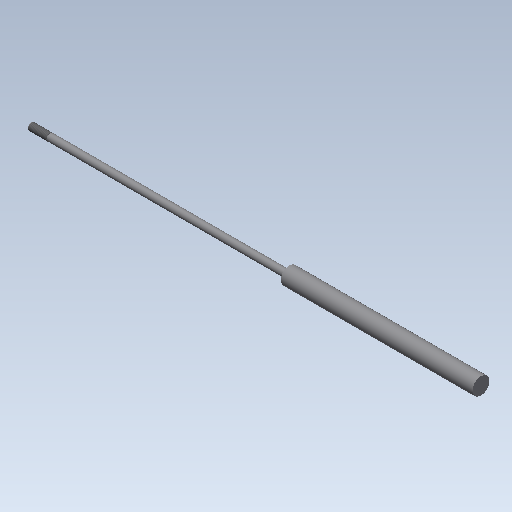
# Autodesk Inventor part: 015.5-P0000_rod
Saved by Autodesk Inventor 2020 (Build 240168000, 168)
## iProperties
Created: 2020-01-07
Part Number: 015.5-P0000_rod
Material: Generic
Catalog Web Link: www.cadenas.de
Description: Standard Air Cylinder_rod-Original Line - Standard Air Cylinders
Vendor: BIMBA
Document SubType Name: Modeling
Designer: psadmin
Manufacturer: BIMBA
Mass: 15.5246 g
Surface Area: 71.9082 cm^2
Volume: 15.5246 cm^3
Density: 1 g/cm^3
Appearance: PSOLRGB-181-181-181
Category: PARTsolutions
Company: BIMBA
PSOL_IDENT_0: {$CADENAS_DATA\23d-libs\bimba\bimba_brand\bimba_imperial\bimba_full_line\original_line_cylinders\sta
PSOL_IDENT_1: ndard_air_cylinders\rod.prj},331 {VTYP=3D},{NB=015.5-P0000_rod},{LINA=015.5-P0000_rod},{NN=Standard
PSOL_IDENT_2: Air Cylinder_rod},{DATE=23.12.2019 10:36:48},{GEOMDATE=27.08.2019 11:00:52},{VERSION=},{LINEID=30},{
PSOL_IDENT_3: WBVAR=STROKE,ACTING,MNT,DER,NR,BM,CO,M,EE,EEL,K,Q,Y,F,G,T,B,H,SER,SR,NT,W,E,HL,ST,STP,PRC,PB,COLOR1,
PSOL_IDENT_4: FCD,RCD,BCD,ZHJ},{WBNUMERIC=STROKE,EEL,COLOR1,FCD,RCD,BCD,ZHJ}  {NB=015.5-P0000_rod},{LINA=015.5-P00
PSOL_IDENT_5: 00_rod},{KT=DUMMY},{PN=015.5-P000},{DASH=-},{BORE=0.43750000},{BOREPN=01},{STROKE=5.500},{STROKEALG=
PSOL_IDENT_6: [0.001:50/0.001]},{STROKE1=5.500},{ACTING=},{ACTINGALG= '' , 'Single Acting' , 'R' , 'Reverse Single
PSOL_IDENT_7: Acting' , 'D' , 'Double Acting' },{ACTINGPN=},{MNT=P},{MNTALG= '' , 'Front Nose Mounting' , 'P' , '
PSOL_IDENT_8: Rear Pivot Mounting' , 'BF' , 'Front Block Mounting' , 'BR' , 'Rear Block Mounting for Vertical Posi
PSOL_IDENT_9: tioning' , 'BFT' , 'Front Block Trunnion Mounting' , 'BRT' , 'Rear Block Trunnion Mounting' },{TYPE=
PSOL_IDENT_10: },{MNTPN=P},{DER=},{DERALG= '' , 'N/A' },{NR=},{NRALG= '' , 'Standard' , 'NR' , 'Non-rotating - Hexa
PSOL_IDENT_11: gon Rod' },{NRPN=},{BM=},{BMALG= '' , 'N/A' },{BMPN=},{CO=},{COALG= '' , 'N/A' },{M=},{MALG= '', 'Wi
PSOL_IDENT_12: thout Magnet', 'M', 'With Magnet' },{EE=},{EEL=0},{EEMAX=44},{EEALG= '', 'Without Extra Extension', '
PSOL_IDENT_13: EE', 'With Extra Extension' },{EELALG=0},{EEPN=},{EEPN1=0.000},{K=},{KALG= '', 'Standard' , 'K' , 'P
PSOL_IDENT_14: orts Rotated 90deg' },{KPN=},{Q=},{QALG= '' , 'Without Side Ported Rear Head' , 'Q' , 'With Side Por
PSOL_IDENT_15: ted Rear Head' },{QPN=},{Y=},{YALG= '' , 'Without Pivot Bushing' , 'Y' , 'With Pivot Bushing' },{YPN=
PSOL_IDENT_16: },{F=},{FALG= '', 'Standard', 'F', 'Molycoated Body' },{FPN=},{G=},{GPN=},{T=},{TALG= '' , 'Standard'
PSOL_IDENT_17: , 'N' , 'Low Temperature' , 'V' , 'High Temperature' },{NPN=},{VPN=},{B=},{BALG= '', 'Without Bumpe
PSOL_IDENT_18: r' , 'B' , 'With Bumper' },{BPN=},{H=},{HALG= '', 'N/A' },{HPN=},{SER=},{SERALG= '' , 'N/A' },{SR=},
PSOL_IDENT_19: {SRALG= 'C' , 'Carbon Steel Rod' , 'SR' , '303 Stainless Steel Rod' , '' , '303 Stainless Steel Rod1'
PSOL_IDENT_20: },{SRPN=},{SRCON=0},{NT=},{NTPN=},{W=},{WALG= '' , 'N/A' },{WPN=},{E=},{EALG= '' , 'Without Special
PSOL_IDENT_21: Lube and Seals' , 'E' , 'With Special Lube and Seals' },{EPN=},{HL=},{HLALG= '' , 'N/A' },{ST=},{ST
PSOL_IDENT_22: ALG= '' , 'Without Switch Track' , 'T' , 'With Switch Track' },{STP=},{STPALG= '' , 'N/A' },{STPN=},
PSOL_IDENT_23: {PRC=},{PRCALG= '' , 'Without Piston Rod Clevis' , 'D-166-1' , 'With Piston Rod Clevis' },{PRCPN=},{
PSOL_IDENT_24: PB=},{PBALG= '' , 'Without Pivot Bracket' , 'D-167' , 'With Pivot Bracket' },{PBPN=},{TLEN=10.8620},
PSOL_IDENT_25: {TEXT=0.466667},{SPACE=0.266667},{FRAC=12.0900},{RGCON=},{RGDACCON=},{RHCON=P},{RHCONON=1},{RHACCON=
PSOL_IDENT_26: },{FNUTCON=0},{RNUTCON=0},{FNUTPN=},{RNUTPN=},{FNUTTRANS=0.0000},{RNUTTRANS=0.0000},{VHOLECON=2},{A1=
PSOL_IDENT_27: 0.6880},{A1N=0.6880},{A1P=1.1880},{A1B=1.1880},{A4=0.2500},{A4N=0.2500},{A4P=0.1880},{A5=0.0200},{A1
PSOL_IDENT_28: H=1.188},{A1NH=0.5000},{A1PH=1.1880},{A1BH=0.8120},{A1SH=0.0000},{A2H=0.1880},{A2NH=0.1880},{LENGTH=
PSOL_IDENT_29: 1.7500},{LENGTH1=1.7500},{LENGTH2=2.6100},{MUL=10.3400},{MUL11=10.3400},{MUL22=15.8400},{MUL33=10.34
PSOL_IDENT_30: 00},{MUL2=0.9400},{MUL211=0.9400},{MUL222=1.4400},{MUL233=0.9400},{SSS=11.0000},{RGLEN=0.4580},{RHLE
PSOL_IDENT_31: N=0.7700},{SSS1=11.0000},{A13=0.9380},{THDLEN1=0.5000},{THD1=0.1900},{TAB=UNF},{THDLEN=0.5000},{THD=
PSOL_IDENT_32: 0.1900},{OD=0.4465},{RODL=11.6520},{PL=4.9640},{RODDIA=0.1870},{HEX=0.1870},{RODTRANS=0.0000},{G1=0.
PSOL_IDENT_33: 0000},{ON=0},{G5=0.0000},{DERLEN=6.6880},{THOLE=0.0000},{WF=0.0000},{BADD=0.0000},{MADD=0.0000},{NVA
PSOL_IDENT_34: DD=0.000},{JRADD=0.00000},{COLOR=0.71,0.71,0.71,0.00},{GROOVE=1},{HOL=0},{D7=0.1590},{H1=0.0000},{D1=
PSOL_IDENT_35: 0.4840},{D1RH=0.7380},{D1P=0.0000},{D1B=0.7380},{D1N=0.4840},{D1NRH=0.4855},{D1BRH=0.4855},{D1PRH=0.
PSOL_IDENT_36: 7380},{BOZO=1},{HADD=0.000},{COLOR1=0},{DEFL=0.0000},{HEXL=0.0000},{SSADD=0.0000},{WFL=0.0000},{MOVE=
PSOL_IDENT_37: 0.0000},{PRCL2=0.37500},{PRCB=0.12000},{PRCTRANS=0.00000},{FCD=0},{RCD=0},{BCD=0},{ZHJ=0.000}
NN: Standard Air Cylinder_rod
NT: Standard
NB: 015.5-P0000_rod
NBSYN: $PN.$COLOR1._rod
LINA: 015.5-P0000_rod
PN: 015.5-P000
BORE: 0.4375
BOREPN: 01
STROKE: 5.5
ACTING: Single Acting
MNT: Rear Pivot Mounting
DER: N/A
NR: Standard
BM: N/A
CO: N/A
M: Without Magnet
EE: Without Extra Extension
EEL: 0
K: Standard
Q: Without Side Ported Rear Head
Y: Without Pivot Bushing
F: Standard
G: Without Magnalube Lubrication
T: Standard
B: Without Bumper
H: N/A
SER: N/A
SR: 303 Stainless Steel Rod1
W: N/A
E: Without Special Lube and Seals
HL: N/A
ST: Without Switch Track
STP: N/A
PRC: Without Piston Rod Clevis
PB: Without Pivot Bracket
A1N: 0.688
A1P: 1.188
A1B: 1.188
A4N: 0.25
A4P: 0.188
A5: 0.02
A1NH: 0.5
A1PH: 1.188
A1BH: 0.812
A1SH: 0
A2NH: 0.188
A13: 0.938
THDLEN1: 0.5
THD1: 0.19
TAB: UNF
OD: 0.4465
RODDIA: 0.187
HEX: 0.187
G1: 0
G5: 0
THOLE: 0
WF: 0
GROOVE: 1
D7: 0
D1P: 0
D1B: 0.738
D1N: 0.484
D1NRH: 0.4855
D1BRH: 0.4855
D1PRH: 0.738
COLOR1: 0
FCD: 0
RCD: 0
BCD: 0
ZHJ: 0
SUPPLIER: BIMBA
ARTICLENO: 015.5-P0000_rod
BOMINFO: 015.5-P0000_rod
CREATOR: CADENAS GmbH
d5: 0.000 in
d6: 0.000 in
d8: 0.000 in
d9: 0.000 in
d10: 0.000 in
Title: 015.5-P0000_rod
Author: Cadenas PARTsolutions
Comments: Original Line - Standard Air Cylinders
Autodesk Inventor part; units mm, degrees
sketch "Sketch_1" plane through (0, 0, 0) normal (0, 0, 1) x (1, 0, 0)
  line L0 (283.2608, 0) -> (0, 0)
  line L1 (0, 0) -> (0, 2.3749)
  line L2 (0, 2.3749) -> (157.1752, 2.3749)
  line L3 (157.1752, 2.3749) -> (157.1752, 5.6197)
  line L4 (157.1752, 5.6197) -> (283.2608, 5.6197)
  line L5 (283.2608, 5.6197) -> (283.2608, 0)
  line L6 (283.2608, 0) -> (0, 0)
  constraints: 14 end point
revolve "Revolution1" add sketch "Sketch_1" angle 360 about axis through (283.2608, 0, 0) along (1, 0, 0)
sketch "Sketch_3" plane through (0, 0, 0) normal (0, 0, 1) x (1, 0, 0)
  line L0 (0, 0) -> (-12.7, 0)
  line L1 (-12.7, 0) -> (-12.7, 1.9406)
  line L2 (-12.7, 1.9406) -> (-12.2276, 2.413)
  line L3 (-12.2276, 2.413) -> (0, 2.413)
  line L4 (0, 2.413) -> (0, 0)
  line L5 (0, 0) -> (-12.7, 0)
  constraints: 12 end point
revolve "Revolution2" add sketch "Sketch_3" angle 360 about axis through (0, 0, 0) along (1, 0, 0)
thread "Thread1" size "10-32 UNF" class "2A" standard "ANSI Unified Screw Threads" full length
sketch "Sketch_30" plane through (0, 0, 0) normal (0, 0, 1) x (1, 0, 0)
  line L0 (0, 0) -> (-0.254, 0)
  line L1 (-0.254, 2.159) -> (0, 2.159)
  line L2 (0, 2.159) -> (0, 2.667)
  line L3 (0, 2.667) -> (-0.254, 2.667)
  line L4 (-0.254, 2.667) -> (-0.254, 2.159)
  constraints: 10 end point
revolve "Revolution3" cut sketch "Sketch_30" angle 360 about axis through (0, 0, 0) along (1, 0, 0)
ref_plane "dia1_XY" through (0, 2.3749, 0) normal (1, 0, 0) x (0, 0, -1)
ref_plane "dia1_YZ" through (0, 2.3749, 0) normal (0, 0, -1) x (0, 1, 0)
ref_plane "dia1_ZX" through (0, 2.3749, 0) normal (0, 1, 0) x (1, 0, 0)
ref_plane "dia12_XY" through (0, 0, 6.1468) normal (1, 0, 0) x (0, 0, -1)
ref_plane "dia12_YZ" through (0, 0, 6.1468) normal (0, 0, -1) x (0, 1, 0)
ref_plane "dia12_ZX" through (0, 0, 6.1468) normal (0, 1, 0) x (1, 0, 0)
ref_plane "dia1r_XY" through (0, 0, 9.3726) normal (1, 0, 0) x (0, 0, -1)
ref_plane "dia1r_YZ" through (0, 0, 9.3726) normal (0, 0, -1) x (0, 1, 0)
ref_plane "dia1r_ZX" through (0, 0, 9.3726) normal (0, 1, 0) x (1, 0, 0)
ref_plane "dia2_XY" through (0, -2.3749, 0) normal (1, 0, 0) x (0, 0, -1)
ref_plane "dia2_YZ" through (0, -2.3749, 0) normal (0, 0, -1) x (0, 1, 0)
ref_plane "dia2_ZX" through (0, -2.3749, 0) normal (0, 1, 0) x (1, 0, 0)
ref_plane "dia22_XY" through (0, 0, -6.1468) normal (1, 0, 0) x (0, 0, -1)
ref_plane "dia22_YZ" through (0, 0, -6.1468) normal (0, 0, -1) x (0, 1, 0)
ref_plane "dia22_ZX" through (0, 0, -6.1468) normal (0, 1, 0) x (1, 0, 0)
ref_plane "dia2r_XY" through (0, 0, -9.3726) normal (1, 0, 0) x (0, 0, -1)
ref_plane "dia2r_YZ" through (0, 0, -9.3726) normal (0, 0, -1) x (0, 1, 0)
ref_plane "dia2r_ZX" through (0, 0, -9.3726) normal (0, 1, 0) x (1, 0, 0)
ref_plane "rl1_XY" through (-12.7, 0, 0) normal (1, 0, 0) x (0, 0, -1)
ref_plane "rl1_YZ" through (-12.7, 0, 0) normal (0, 0, -1) x (0, 1, 0)
ref_plane "rl1_ZX" through (-12.7, 0, 0) normal (0, 1, 0) x (1, 0, 0)
ref_plane "rl2_XY" through (0, 0, 0) normal (1, 0, 0) x (0, 0, -1)
ref_plane "rl2_YZ" through (0, 0, 0) normal (0, 0, -1) x (0, 1, 0)
ref_plane "rl2_ZX" through (0, 0, 0) normal (0, 1, 0) x (1, 0, 0)
ref_plane "rod_cp_XY" through (0, 0, 0) normal (1, 0, 0) x (0, 0, -1)
ref_plane "rod_cp_YZ" through (0, 0, 0) normal (0, 0, -1) x (0, 1, 0)
ref_plane "rod_cp_ZX" through (0, 0, 0) normal (0, 1, 0) x (1, 0, 0)
ref_plane "thd1_XY" through (-12.7, 2.413, 0) normal (1, 0, 0) x (0, 0, -1)
ref_plane "thd1_YZ" through (-12.7, 2.413, 0) normal (0, 0, -1) x (0, 1, 0)
ref_plane "thd1_ZX" through (-12.7, 2.413, 0) normal (0, 1, 0) x (1, 0, 0)
ref_plane "thd2_XY" through (-12.7, -2.413, 0) normal (1, 0, 0) x (0, 0, -1)
ref_plane "thd2_YZ" through (-12.7, -2.413, 0) normal (0, 0, -1) x (0, 1, 0)
ref_plane "thd2_ZX" through (-12.7, -2.413, 0) normal (0, 1, 0) x (1, 0, 0)
ref_plane "to_rod_clevis_XY" through (-12.7, 0, 0) normal (1, 0, 0) x (0, 0, -1)
ref_plane "to_rod_clevis_YZ" through (-12.7, 0, 0) normal (0, 0, -1) x (0, 1, 0)
ref_plane "to_rod_clevis_ZX" through (-12.7, 0, 0) normal (0, 1, 0) x (1, 0, 0)
body "Solid1"
